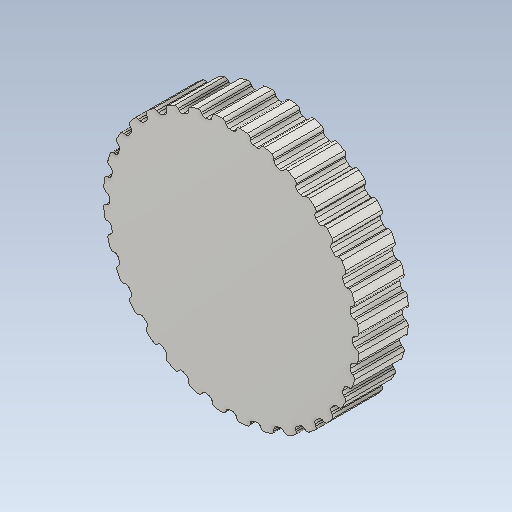
# Autodesk Inventor part: Синхронный шкив3
Saved by Autodesk Inventor 2021 (Build 250183000, 183)
## iProperties
Created: 2021-06-16
Part Number: Синхронный шкив3
Material: Steel
Document SubType Name: Modeling
Designer: panda
Density: 1 g/cm^3
Appearance: Steel
CustomPartVersion: 1
Author: panda
Autodesk Inventor part; units mm, degrees
ref_plane "YZ Plane" through (0, 0, 0) normal (1, 0, 0) x (0, 1, 0)
ref_plane "XZ Plane" through (0, 0, 0) normal (0, 1, 0) x (-1, 0, 0)
ref_plane "XY Plane" through (0, 0, 0) normal (0, 0, 1) x (1, 0, 0)
sketch "Эскиз шкива" plane through (0, 0, 0) normal (0, 0, 1) x (1, 0, 0)
  circle A0 centre (0, 0) radius 64.6806 construction
  circle A1 centre (0, 0) radius 63.9948
  circle A2 centre (0, 0) radius 60.9468
  line L0 (-3.1762, 63.9159) -> (-2.0955, 60.9468)
  line L1 (-2.0955, 60.9468) -> (2.0955, 60.9468)
  line L2 (2.0955, 60.9468) -> (3.1762, 63.9159)
  line L3 (0, 0) -> (0, 63.9948) construction
  point P0 (0, 60.9468)
  dimension "d0" = 129.3611
  dimension "d1" = 0.6858
  dimension "d2" = 3.048
  dimension "d3" = 40
  dimension "d4" = 4.191
  constraints: 8 end point, 3 coincident, 3 point on circle, 2 centre point, 1 horizontal, 1 midpoint, 1 point on line, 1 vertical, 1 vertical alignment, 3 other
  measures "d0" diameter of A0
  measures "d1" radial gap between concentric circles of A0 A1
  measures "d3" angle of L2 L0
  measures "d4" distance of L0.end L1.end
extrude "Базовое тело" add sketch "Эскиз шкива" along normal mid plane 24.892 contours A2 | A1 L0 L1 L2 | L2 L1 L0 A1
extrude "Зуб" cut sketch "Эскиз шкива" along normal through all both and the other way through all contours L2 L1 L0 A1 picked at (0, 62.973)
fillet "Fillet" radius 1.6002 2 edges at (2.0955, 60.9468, 0) (-2.0955, 60.9468, 0)
fillet "Fillet" radius 1.6002 4 edges at (-3.1762, 63.9159, 6.223) (-3.1762, 63.9159, -6.223) (3.1762, 63.9159, 6.223) (3.1762, 63.9159, -6.223)
pattern_circular "Зубья" count 32 over 360 about axis through (0, 0, -10) along (0, 0, 1) of "Зуб", "Fillet"
feature "Левый фланец" [suppressed]
feature "Правый фланец" [suppressed]
equation "\"d1\" = da_a"
equation "\"d2\" = da_hg"
equation "\"d3\" = 2 * da_fi"
equation "\"d4\" = da_bw"
equation "\"d5\" = da_bf"
equation "\"d7\" = da_bf"
equation "\"d9\" = da_rb"
equation "\"d10\" = da_rt"
equation "\"da_pb\" = 12.7"
equation "\"da_fi\" = 20deg"
equation "\"da_hg\" = 3.048"
equation "\"da_bw\" = 4.191"
equation "\"da_rb\" = 1.6002"
equation "\"da_rt\" = 1.6002"
equation "\"da_a\" = 0.6858"
equation "\"da_bf\" = 24.892"
equation "\"da_wf\" = 1.5"
equation "\"da_hf\" = 1.5"
body "Solid1"
